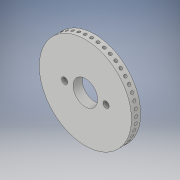
# Autodesk Inventor part: Крепление
Saved by Autodesk Inventor 2017 (Build 210142000, 142)
## iProperties
Part Number: Крепление
Material: Типовые
Document SubType Name: Modeling
Designer: Daemon
Density: 1 g/cm^3
Appearance: По умолчанию
Author: Daemon
Autodesk Inventor part; units mm, degrees
ref_plane "XZ Plane" through (0, 0, 0) normal (0, 1, 0) x (-1, 0, 0)
ref_plane "XY Plane" through (0, 0, 0) normal (0, 0, 1) x (1, 0, 0)
sketch "Эскиз1" plane through (0, 0, 0) normal (0, 0, 1) x (1, 0, 0)
  circle A0 centre (0, 0) radius 4
  circle A1 centre (0, 0) radius 15
  dimension "d0" = 8
  dimension "d2" = 30
  constraints: 2 centre point, 1 coincident
  measures "d0" diameter of A0
  measures "d2" diameter of A1
extrude "Выдавливание1" add sketch "Эскиз1" along normal blind 3
sketch "Эскиз2" plane through (0, 0, 3) normal (0, 0, 1) x (1, 0, 0)
  circle A0 centre (0, 0) radius 6.75
  circle A1 centre (6.75, 0) radius 1
  dimension "d5" = 13.5
  dimension "d6" = 2
  constraints: 1 centre point, 1 coincident, 1 horizontal alignment, 2 other
  measures "d6" diameter of A1
extrude "Выдавливание2" cut sketch "Эскиз2" against normal up to next contours A0 A1 | A0 A1 picked at (6.4242, -0.1935) picked at (7.0444, -0.2621)
pattern_circular "Круговой массив1" count 2 over 360 about axis through (0, 0, 0) along (0, 0, 1) of "Выдавливание2"
ref_plane "РабПлоскость1" through (15, 0, 0) normal (1, 0, 0) x (0, 1, 0)
sketch "Эскиз4" plane through (15, 0, 0) normal (1, 0, 0) x (0, 1, 0)
  line L0 (0, 0) -> (0, 1.5)
  circle A0 centre (0, 1.5) radius 0.5
  dimension "d19" = 1.5
  dimension "d20" = 1
  constraints: 2 end point, 1 centre point, 1 coincident, 1 vertical
  measures "d19" distance of L0.start L0.end
  measures "d20" diameter of A0
extrude "Выдавливание4" cut sketch "Эскиз4" against normal blind 3
pattern_circular "Круговой массив3" count 45 over 360 about axis through (0, 0, 0) along (0, 0, 1) of "Выдавливание4"
